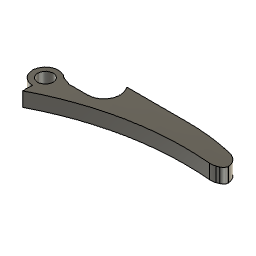
Finger1Section3P1V1 v2 (Autodesk Fusion 360 design; units mm, degrees)
Autodesk Fusion 360 part; units mm, degrees
sketch "Sketch1" plane through (0, 0, 0) normal (0, 0, 1) x (1, 0, 0)
  circle A0 centre (0.507, 0) radius 1.2
  line L0 (8.001, 5) -> (17.4161, 5)
  arc A1 (1.9212, 1.4142) -> (0.507, -2) centre (0.507, 0) ccw
  line L1 (0.507, -2) -> (0.507, -3.5)
  arc A2 (24.488, 1.2302) -> (0.507, -3.5) centre (20.507, -41.7412) ccw
  line L2 (37.507, -0.5557) -> (37.507, -2.0752)
  line L3 (3.2141, 0.937) -> (6.0466, 0.937)
  line L4 (3.2141, 0.937) -> (1.9212, 1.4142)
  arc A3 (6.0466, 0.937) -> (8.001, 5) centre (6.0466, 3.4386) ccw
  line L5 (23.6345, 4.3484) -> (24.5233, 4.1601)
  line L6 (26.3774, 2.9193) -> (26.3838, 2.91)
  line L7 (26.3838, 2.1013) -> (26.3838, 2.346)
  arc A4 (23.6345, 4.3484) -> (17.4161, 5) centre (17.4161, -25) ccw
  arc A5 (25.3483, 3.8533) -> (24.5233, 4.1601) centre (23.9015, 1.2253) ccw
  arc A6 (26.3838, 2.1013) -> (25.3483, 3.8533) centre (24.3838, 2.1013) ccw
  line L8 (25.791, 1.5001) -> (25.3553, 1.3418)
  arc A7 (25.791, 1.5001) -> (26.3838, 2.346) centre (25.4838, 2.346) ccw
  arc A8 (24.488, 1.2302) -> (25.3553, 1.3418) centre (24.6725, 3.2217) ccw
  dimension "d3" = 2.4
  dimension "d7" = 4
  dimension "d10" = 1.5
  dimension "d15" = 30
  dimension "d16" = 3
  dimension "d17" = 2
  dimension "d18" = 0.9
  dimension "d19" = 2
  constraint concentric A0 A1
  constraint tangent L3 A3
  constraint vertical L7
  constraint tangent L0 A4
  constraint tangent L5 A4
  constraint tangent L5 A5
  constraint tangent L6 A5
  constraint tangent A5 A6
  constraint tangent L7 A6
  constraint tangent L8 A7
  constraint tangent L7 A7
  constraint tangent A2 A8
  constraint tangent L8 A8
  measures "d3" diameter of A0
  measures "d7" diameter of A1
  measures "d10" distance of L1.end A1.end
  measures "d15" radius of A4
  measures "d16" radius of A5
  measures "d17" radius of A6
  measures "d18" radius of A7
  measures "d19" radius of A8
extrude "Extrude2" add sketch "Sketch1" along normal blind 2.2 contours L0 A1 L1 A2 L3 L4 A3 L5 A4 A5 A6 L8 A7 A8
